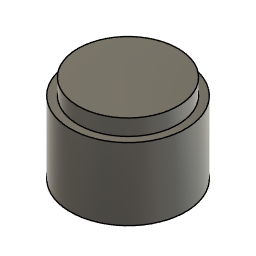
rotating_holder (Autodesk Fusion 360 archive; units mm, degrees)
design "ultrasonic_sensor"
Autodesk Fusion 360 part; units mm, degrees
sketch "Sketch1" plane through (0, 0, 0) normal (0, 1, 0) x (1, 0, 0)
  circle A0 centre (0, 0) radius 7.2
  circle A1 centre (0, 0) radius 6.25
  dimension "d1" = 14.4
  dimension "d2" = 12.5
  constraint coincident A0.centre A1.centre
  measures "d1" diameter of A0
  measures "d2" diameter of A1
extrude "Extrude1" add sketch "Sketch1" along normal blind 9 contours A0 | A1
extrude "Extrude2" add sketch "Sketch1" along normal blind 2 from surface at 9 contours A1
